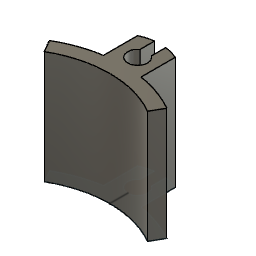
bowden_cable_guide_finger (Autodesk Fusion 360 design; units mm, degrees)
Autodesk Fusion 360 part; units mm, degrees
sketch "Sketch1" plane through (0, 0, 0) normal (0, 1, 0) x (1, 0, 0)
  circle A0 centre (0, 0) radius 11
  circle A1 centre (0, 0) radius 12.5
  line L0 (0, 0) -> (9.5756, 8.0348)
  line L1 (0, 0) -> (12.5, 0) construction
  line L2 (0, 0) -> (-9.5756, 8.0348)
  line L3 (0, 0) -> (12.5, 0) construction
  line L4 (0, 0) -> (-4.7878, 11.5467)
  line L5 (-4.7878, 11.5467) -> (4.7878, 11.5467)
  circle A2 centre (0, 11.5467) radius 4.8552
  line L6 (0, 11.5467) -> (0, 16.402)
  circle A3 centre (0, 13.9744) radius 1.05
  circle A4 centre (0, 13.9744) radius 0.5
  line L7 (0, 16.402) -> (-0.6, 16.402)
  line L8 (0, 16.402) -> (0.6, 16.402)
  line L9 (-0.6, 16.402) -> (-0.6, 14.836)
  line L10 (0.6, 16.402) -> (0.6, 14.836)
  line L11 (0, 0) -> (6.25, 10.8253)
  line L12 (0, 0) -> (12.5, 0) construction
  line L13 (0, 0) -> (-6.25, 10.8253)
  line L14 (0, 11.5467) -> (2, 11.5467)
  line L15 (0, 11.5467) -> (-2, 11.5467)
  line L16 (2, 11.5467) -> (-2, 11.5467)
  line L17 (-2, 11.5467) -> (-2, 15.9709)
  line L18 (-2, 15.9709) -> (2, 15.9709)
  line L19 (2, 15.9709) -> (2, 11.5467)
  dimension "d1" = 22
  dimension "d2" = 25
  dimension "d3" = 40
  dimension "d4" = 140
  dimension "d5" = 2.1
  dimension "d6" = 1
  dimension "d7" = 0.6
  dimension "d8" = 0.6
  dimension "d9" = 60
  dimension "d10" = 120
  dimension "d13" = 2
  dimension "d14" = 2
  dimension "d15" = 9.5756
  dimension "d16" = 4.4242
  constraint coincident A0.centre A1.centre
  constraint horizontal L1
  constraint horizontal L3
  constraint coincident A1 L4.end
  constraint coincident A1 L5.end
  constraint horizontal L5
  constraint midpoint L5 A2.centre
  constraint coincident A2.centre L6.start
  constraint coincident A2 L6.end
  constraint perpendicular L5 L6
  constraint midpoint L6 A3.centre
  constraint concentric A3 A4
  constraint perpendicular L6 L7
  constraint perpendicular L6 L8
  constraint coincident A3 L9.end
  constraint perpendicular L7 L9
  constraint coincident A3 L10.end
  constraint perpendicular L8 L10
  constraint horizontal L12
  constraint coincident A1 L11.end
  constraint perpendicular L6 L14
  constraint perpendicular L6 L15
  constraint horizontal L16
  constraint vertical L17
  constraint horizontal L18
  constraint vertical L19
  constraint coincident A2 L17.end
  measures "d1" diameter of A0
  measures "d2" diameter of A1
  measures "d3" angle of L0 L1
  measures "d4" angle of L2 L3
  measures "d5" diameter of A3
  measures "d6" diameter of A4
  measures "d7" distance of L6.end L7.end
  measures "d8" distance of L6.end L8.end
  measures "d9" angle of L11 L12
  measures "d10" angle of L11 L13
  measures "d13" distance of A2.centre L14.end
  measures "d14" distance of A2.centre L15.end
  measures "d15" distance of L4.end L5.end
  measures "d16" distance of L14.end L18.end
extrude "Extrude1" add sketch "Sketch1" along normal blind 12 contours A0 A1 A2 L11 | A0 A1 A2 L13 | A0 A1 L4 L5 A2 L14 L15 L16 | A0 A1 L4 A2 | A1 L5 L17 | A1 L5 L19 | A1 L6 A3 L9 L17 L18 | A2 L9 L18 | A1 L5 L6 L15 L16 L17 | A1 L5 L6 L14 L16 L19 | A1 L6 A3 L10 L18 L19 | A2 L10 L18
sketch "Sketch2" plane through (0, 0, 0) normal (0, -1, 0) x (1, 0, 0)
  line L0 (0.6, -14.836) -> (0.6, -16.3648)
  arc A0 (0.6, -16.3648) -> (2, -15.9709) centre (0, -11.5467) ccw
  line L1 (2, -15.9709) -> (2, -12.339)
  arc A1 (2, -12.339) -> (6.25, -10.8253) centre (0, 0) ccw
  line L2 (6.25, -10.8253) -> (5.5, -9.5263)
  arc A2 (-5.5, -9.5263) -> (5.5, -9.5263) centre (0, 0) ccw
  line L3 (-5.5, -9.5263) -> (-6.25, -10.8253)
  arc A3 (-6.25, -10.8253) -> (-2, -12.339) centre (0, 0) ccw
  line L4 (-2, -12.339) -> (-2, -15.9709)
  arc A4 (-2, -15.9709) -> (-0.6, -16.3648) centre (0, -11.5467) ccw
  line L5 (-0.6, -16.3648) -> (-0.6, -14.836)
  arc A5 (0.6, -14.836) -> (-0.6, -14.836) centre (0, -13.9744) ccw
  line L6 (0, -11) -> (0, -12.9244)
  constraint midpoint A2 L6.start
  constraint midpoint A5 L6.end
